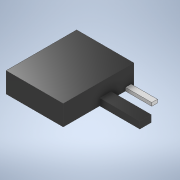
# Autodesk Inventor part: NVidia
Saved by Autodesk Inventor 2021 (Build 250183000, 183)
## iProperties
Created: 2021-02-21
Part Number: NVidia
Material: Generic
Document SubType Name: Modeling
Designer: deuts
Density: 1 g/cm^3
Appearance: Default
Author: deuts
Autodesk Inventor part; units mm, degrees
ref_plane "YZ Plane" through (0, 0, 0) normal (1, 0, 0) x (0, 1, 0)
ref_plane "XZ Plane" through (0, 0, 0) normal (0, 1, 0) x (-1, 0, 0)
ref_plane "XY Plane" through (0, 0, 0) normal (0, 0, 1) x (1, 0, 0)
sketch "Sketch1" plane through (0, 0, 0) normal (0, 1, 0) x (-1, 0, 0)
  line L0 (-40.5, 50) -> (40.5, 50)
  line L1 (40.5, 50) -> (40.5, -50)
  line L2 (40.5, -50) -> (-40.5, -50)
  line L3 (-40.5, -50) -> (-40.5, 50)
  line L4 (-40.5, 50) -> (40.5, -50) construction
  line L5 (40.5, 50) -> (-40.5, -50) construction
  point P0 (0, 0)
  dimension "d0" = 81
  dimension "d1" = 100
  constraints: 12 end point, 2 midpoint, 2 parallel, 1 horizontal, 1 perpendicular
  measures "d0" distance of L1.end L2.end
  measures "d1" distance of L0.end L1.end
extrude "Extrusion1" add sketch "Sketch1" along normal blind 28.7
sketch "Sketch2" plane through (40.5, 0, 50) normal (1, 0, 0) x (0, 0, -1)
  line L0 (100, 0) -> (0, 0) projected
  line L1 (67.9, 0) -> (67.9, 9.6)
  line L2 (67.9, 9.6) -> (51.7, 9.6)
  line L3 (51.7, 9.6) -> (51.7, 0)
  line L4 (51.7, 0) -> (67.9, 0)
  point P0 (50, 0)
  dimension "d5" = 9.6
  dimension "d6" = 16.2
  constraints: 8 end point, 2 perpendicular, 2 point on line, 1 collinear, 1 vertical
  measures "d5" distance of L1.start L1.end
  measures "d6" distance of L1.end L2.end
extrude "Extrusion2" add sketch "Sketch2" along normal blind 56.9
sketch "Sketch3" plane through (40.5, 0, -50) normal (1, 0, 0) x (0, 0, -1)
  line L0 (-32.1, 0) -> (0, 0) projected
  line L1 (0, 0) -> (-3.8, 0)
  line L2 (-3.8, 0) -> (-3.8, 4.6)
  line L3 (-3.8, 4.6) -> (-11.9, 4.6)
  line L4 (-11.9, 4.6) -> (-11.9, 0)
  line L5 (-11.9, 0) -> (-3.8, 0)
  point P0 (-50, 0)
  dimension "d9" = 3.8
  dimension "d10" = 4.6
  dimension "d11" = 8.1
  constraints: 10 end point, 2 perpendicular, 2 point on line, 1 collinear, 1 vertical
  measures "d9" distance of L0.end L1.end
  measures "d10" distance of L1.end L2.end
  measures "d11" distance of L2.end L3.end
extrude "Extrusion3" add sketch "Sketch3" along normal blind 37.4
body "Solid1"
